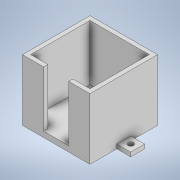
# Autodesk Inventor part: Caixa Motor Definitiva
Saved by Autodesk Inventor 2021 (Build 250183000, 183)
## iProperties
Created: 2021-04-22
Part Number: Caixa Motor Definitiva
Material: Genérico
Document SubType Name: Modeling
Designer: Marc
Density: 1 g/cm^3
Appearance: Valor por defecto
Author: Marc
## iProperties of the stored document _3DPrint.ipt
Created: 2021-04-26
Part Number: _3DPrint
Material: Genérico
Document SubType Name: Modeling
Designer: Marc
Density: 1 g/cm^3
Appearance: Valor por defecto
Author: Marc
Autodesk Inventor part; units mm, degrees
ref_plane "YZ Plane" through (0, 0, 0) normal (1, 0, 0) x (0, 1, 0)
ref_plane "XZ Plane" through (0, 0, 0) normal (0, 1, 0) x (-1, 0, 0)
ref_plane "XY Plane" through (0, 0, 0) normal (0, 0, 1) x (1, 0, 0)
sketch "Boceto1" plane through (0, 0, 0) normal (0, 0, 1) x (1, 0, 0)
  line L0 (-24.25, -22) -> (24.25, -22)
  line L1 (24.25, -22) -> (24.25, 22)
  line L2 (24.25, 22) -> (-24.25, 22)
  line L3 (-24.25, 22) -> (-24.25, -22)
  line L4 (-24.25, -22) -> (24.25, 22) construction
  line L5 (24.25, -22) -> (-24.25, 22) construction
  point P0 (0, 0)
  dimension "d0" = 48.5
  dimension "d1" = 44
  constraints: 12 end point, 2 midpoint, 2 parallel, 1 horizontal, 1 perpendicular
  measures "d0" distance of L2.end L1.end
  measures "d1" distance of L1.end L0.end
extrude "Extrusión1" add sketch "Boceto1" along normal blind 48.5
sketch "Boceto2" plane through (-24.25, 22, 0) normal (0, 1, 0) x (1, 0, 0)
  line L0 (3, -3) -> (45.5, -3)
  line L1 (45.5, -3) -> (45.5, -45.5)
  line L2 (3, -45.5) -> (3, -3)
  line L3 (15.25, -45.5) -> (15.25, -48.5)
  line L4 (33.25, -45.5) -> (33.25, -48.5)
  line L5 (45.5, -45.5) -> (33.25, -45.5)
  line L6 (15.25, -45.5) -> (3, -45.5)
  line L7 (15.25, -48.5) -> (33.25, -48.5)
  constraints: 16 end point, 4 parallel, 1 horizontal, 1 perpendicular, 1 vertical
extrude "Extrusión2" cut sketch "Boceto2" against normal blind 40
sketch "Boceto5" plane through (-24.25, -22, 0) normal (0, -1, 0) x (1, 0, 0)
  line L0 (-10, 19.25) -> (0, 19.25)
  line L1 (0, 29.25) -> (-10, 29.25)
  line L2 (-10, 29.25) -> (-10, 19.25)
  line L3 (0, 0) -> (0, 48.5) projected
  line L4 (0, 19.25) -> (0, 29.25)
  line L5 (48.5, 19.25) -> (58.5, 19.25)
  line L6 (58.5, 19.25) -> (58.5, 29.25)
  line L7 (58.5, 29.25) -> (48.5, 29.25)
  line L8 (48.5, 0) -> (48.5, 48.5) projected
  line L9 (48.5, 19.25) -> (48.5, 29.25)
  circle A0 centre (53.5, 24.25) radius 2
  circle A1 centre (-5, 24.25) radius 2
  point P0 (24.25, 0)
  point P1 (0, 24.25)
  point P2 (48.5, 24.25)
  dimension "d15" = 4
  dimension "d16" = 4
  constraints: 16 end point, 4 point on line, 2 centre point, 2 horizontal, 2 midpoint, 2 parallel, 1 perpendicular
  measures "d15" diameter of A0
  measures "d16" diameter of A1
extrude "Extrusión3" add sketch "Boceto5" against normal blind 3
